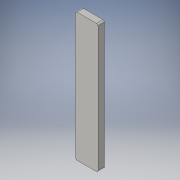
# Autodesk Inventor part: ConnectorRodBodies
Saved by Autodesk Inventor 2016 (Build 200138000, 138)
## iProperties
Created: 2017-03-11
Part Number: ConnectorRodBodies
Material: Generic
Document SubType Name: Modeling
Designer: Owner
Density: 1 g/cm^3
Appearance: Default
Author: Owner
Autodesk Inventor part; units mm, degrees
ref_plane "YZ Plane" through (0, 0, 0) normal (1, 0, 0) x (0, 1, 0)
ref_plane "XZ Plane" through (0, 0, 0) normal (0, 1, 0) x (-1, 0, 0)
ref_plane "XY Plane" through (0, 0, 0) normal (0, 0, 1) x (1, 0, 0)
sketch "Sketch1" plane through (0, 0, 0) normal (0, 0, 1) x (1, 0, 0)
  circle A0 centre (27.1, 34.2286) radius 4 projected
  circle A1 centre (27.1, 34.2286) radius 5 projected
  circle A2 centre (27.0777, 74.6286) radius 4 projected
  circle A3 centre (27.0777, 74.6286) radius 5 projected
  line L0 (32.0777, 105.0354) -> (34.0777, 105.0354)
  line L1 (34.0777, 105.0354) -> (34.0777, 107.0354)
  line L2 (22.0777, 29.2286) -> (20.0777, 29.2286)
  line L3 (20.0777, 29.2286) -> (20.0777, 27.2286)
  line L4 (20.0777, 27.2286) -> (34.0777, 27.2286)
  line L5 (34.0777, 27.2286) -> (34.0777, 107.0354)
  line L6 (34.0777, 107.0354) -> (20.0777, 107.0354)
  line L7 (20.0777, 107.0354) -> (20.0777, 27.2286)
  line L8 (20.0777, 74.6286) -> (20.0777, 34.2286)
  line L9 (22.0777, 100.0373) -> (22.1, 34.2259)
  line L10 (22.1, 100.0373) -> (22.1, 34.2259)
  point P0 (0, 0)
  dimension "d0" = 2
  dimension "d1" = 2
  dimension "d2" = 2
  dimension "d3" = 2
  dimension "d8" = 79.8068
  dimension "d9" = 65.8114
  constraints: 22 end point, 3 horizontal, 3 perpendicular, 2 parallel, 1 point on line
  measures "d0" distance of L0.start L0.end
  measures "d1" distance of L0.end L1.end
  measures "d2" distance of L2.start L2.end
  measures "d3" distance of L2.end L3.end
  measures "d8" distance of L1.end L4.end
  measures "d9" distance of L9.end L9.start
extrude "Extrusion2" add sketch "Sketch1" along normal blind 4 contours A0 | L9 A3 L10 | A1 | L9 A3 L10 | A3 L9 | L10 A3 | A2 | L5 L4 L3 L7 L6 L1
fillet "Fillet1" radius 1 4 edges at (34.0777, 107.0354, 2) (20.0777, 107.0354, 2) (34.0777, 27.2286, 2) (20.0777, 27.2286, 2)
body "Solid2"
